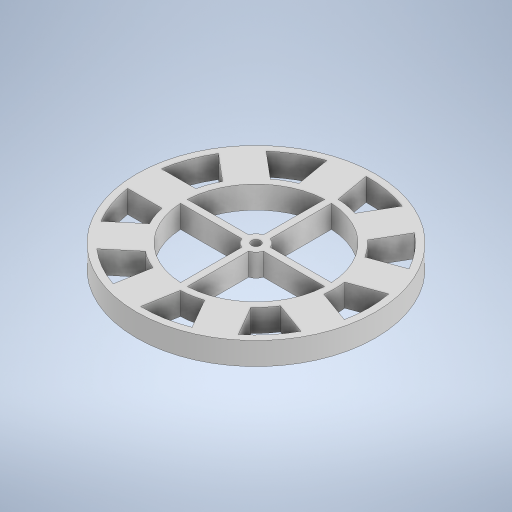
# Autodesk Inventor part: Rueda_SENSORVEL
Saved by Autodesk Inventor 2023 (Build 270158000, 158)
## iProperties
Created: 2022-07-06
Part Number: Rueda_SENSORVEL
Material: Generic
Document SubType Name: Modeling
Designer: franc
Density: 1 g/cm^3
Appearance: Default
Author: franc
Autodesk Inventor part; units mm, degrees
ref_plane "YZ Plane" through (0, 0, 0) normal (1, 0, 0) x (0, 1, 0)
ref_plane "XZ Plane" through (0, 0, 0) normal (0, 1, 0) x (-1, 0, 0)
ref_plane "XY Plane" through (0, 0, 0) normal (0, 0, 1) x (1, 0, 0)
sketch "Sketch1" plane through (0, 0, 0) normal (0, 1, 0) x (-1, 0, 0)
  circle A0 centre (0, 0) radius 50
  circle A1 centre (0, 0) radius 35
  line L0 (49.4343, 7.5) -> (34.187, 7.5)
  line L1 (49.4343, -7.5) -> (34.187, -7.5)
  line L2 (41.8106, 7.5) -> (41.8106, -7.5) construction
  circle A2 centre (0, 0) radius 32
  line L3 (34.187, 7.5) -> (34.187, -7.5)
  line L4 (49.4343, 7.5) -> (49.4343, -7.5)
  line L5 (21.3678, 27.7203) -> (31.0097, 16.2296)
  line L6 (42.6898, 26.0304) -> (31.0097, 16.2296)
  line L7 (33.048, 37.5211) -> (42.6898, 26.0304)
  line L8 (33.048, 37.5211) -> (21.3678, 27.7203)
  line L9 (-1.4496, 34.97) -> (13.3226, 32.3652)
  line L10 (15.9702, 47.3809) -> (13.3226, 32.3652)
  line L11 (1.1981, 49.9856) -> (15.9702, 47.3809)
  line L12 (1.1981, 49.9856) -> (-1.4496, 34.97)
  line L13 (-23.5887, 25.8568) -> (-10.5983, 33.3568)
  line L14 (-18.222, 46.5614) -> (-10.5983, 33.3568)
  line L15 (-31.2123, 39.0614) -> (-18.222, 46.5614)
  line L16 (-31.2123, 39.0614) -> (-23.5887, 25.8568)
  line L17 (-34.6904, 4.6449) -> (-29.5601, 18.7403)
  line L18 (-43.8879, 23.9552) -> (-29.5601, 18.7403)
  line L19 (-49.0182, 9.8598) -> (-43.8879, 23.9552)
  line L20 (-49.0182, 9.8598) -> (-34.6904, 4.6449)
  line L21 (-29.5601, -18.7403) -> (-34.6904, -4.6449)
  line L22 (-49.0182, -9.8598) -> (-34.6904, -4.6449)
  line L23 (-43.8879, -23.9552) -> (-49.0182, -9.8598)
  line L24 (-43.8879, -23.9552) -> (-29.5601, -18.7403)
  line L25 (-10.5983, -33.3568) -> (-23.5887, -25.8568)
  line L26 (-31.2123, -39.0614) -> (-23.5887, -25.8568)
  line L27 (-18.222, -46.5614) -> (-31.2123, -39.0614)
  line L28 (-18.222, -46.5614) -> (-10.5983, -33.3568)
  line L29 (13.3226, -32.3652) -> (-1.4496, -34.97)
  line L30 (1.1981, -49.9856) -> (-1.4496, -34.97)
  line L31 (15.9702, -47.3809) -> (1.1981, -49.9856)
  line L32 (15.9702, -47.3809) -> (13.3226, -32.3652)
  line L33 (31.0097, -16.2296) -> (21.3678, -27.7203)
  line L34 (33.048, -37.5211) -> (21.3678, -27.7203)
  line L35 (42.6898, -26.0304) -> (33.048, -37.5211)
  line L36 (42.6898, -26.0304) -> (31.0097, -16.2296)
  circle A3 centre (0, 0) radius 53
  circle A4 centre (0, 0) radius 2
  circle A5 centre (0, 0) radius 5
  line L37 (1.5, -31.9648) -> (1.5, -4.7697)
  line L38 (-1.5, -31.9648) -> (-1.5, -4.7697)
  line L39 (1.5, -18.3673) -> (-1.5, -18.3673) construction
  line L40 (-31.9648, -1.5) -> (-4.7697, -1.5)
  line L41 (-4.7697, 1.5) -> (-31.9648, 1.5)
  line L42 (1.5, 31.9648) -> (1.5, 4.7697)
  line L43 (-1.5, 4.7697) -> (-1.5, 31.9648)
  line L44 (4.7697, -1.5) -> (31.9648, -1.5)
  line L45 (4.7697, 1.5) -> (31.9648, 1.5)
  line L46 (18.3673, -1.5) -> (18.3673, 1.5) construction
  line L47 (-1.5, 18.3673) -> (1.5, 18.3673) construction
  line L48 (-18.3673, 1.5) -> (-18.3673, -1.5) construction
  point P0 (41.8106, 0)
  point P1 (36.8497, 21.13)
  point P2 (27.2079, 32.6207)
  point P3 (14.6464, 39.8731)
  point P4 (-0.1257, 42.4778)
  point P5 (-14.4101, 39.9591)
  point P6 (-27.4005, 32.4591)
  point P7 (-36.724, 21.3478)
  point P8 (-41.8543, 7.2524)
  point P9 (-41.8543, -7.2524)
  point P10 (-36.724, -21.3478)
  point P11 (-27.4005, -32.4591)
  point P12 (-14.4101, -39.9591)
  point P13 (-0.1257, -42.4778)
  point P14 (14.6464, -39.8731)
  point P15 (27.2079, -32.6207)
  point P16 (36.8497, -21.13)
  point P17 (0, -18.3673)
  point P18 (-34.6904, -4.6449)
  dimension "d0" = 100
  dimension "d1" = 15
  dimension "d2" = 15
  dimension "d3" = 3
  dimension "d6" = 360
  dimension "d8" = 3
  dimension "d9" = 4
  dimension "d11" = 3
  dimension "d12" = 3
  dimension "d13" = 3
  dimension "d14" = 3
  constraints: 98 end point, 12 midpoint, 7 coincident, 5 point on circle, 4 centre point, 4 parallel, 4 point on line, 3 horizontal, 3 vertical, 1 horizontal alignment, 1 perpendicular, 1 vertical alignment, 120 other
  measures "d0" diameter of A0
  measures "d1" radial gap between concentric circles of A0 A1
  measures "d2" distance between parallel lines of L1 L0
  measures "d8" radial gap between concentric circles of A3 A0
  measures "d9" diameter of A4
  measures "d12" distance between parallel lines of L37 L38
  measures "d13" distance between parallel lines of L44 L45
  measures "d14" distance between parallel lines of L43 L42
extrude "Extrusion1" add sketch "Sketch1" along normal blind 10 contours A0 L4 | L4 L1 A1 L0 | L7 A0 | L6 A1 L8 L7 | L3 A1 L33 L29 L25 L21 L17 L13 L9 L5 | A1 L3 | A0 L35 | L35 L34 A1 L36 | L5 A1 | A1 L33 | L11 A0 | L10 A1 L12 L11 | A0 L31 | L31 L30 A1 L32 | L9 A1 | A1 L29 | L15 A0 | L14 A1 L16 L15 | A0 L27 | L27 L26 A1 L28 | L13 A1 | A1 L25 | L19 A0 | L18 A1 L20 L19 | A0 L23 | L23 L22 A1 L24 | L17 A1 | A1 L21 | A2 L44 A5 L45 | L42 A5 L43 A2 | A5 | A2 L38 A5 L37 | L41 A5 L40 A2 | A3 | A4
hole "Hole1" at (0, 0, 0) direction (0, 1, 0) diameter 4 end through all
body "Solid1"
